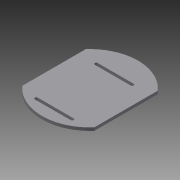
# Autodesk Inventor part: top
Saved by Autodesk Inventor 2015 (Build 190159000, 159)
## iProperties
Created: 2014-10-29
Part Number: top
Material: Generic
Document SubType Name: Modeling
Designer: Colin
Density: 1 g/cm^3
Appearance: Default
Author: Colin
Autodesk Inventor part; units mm, degrees
ref_plane "YZ Plane" through (0, 0, 0) normal (1, 0, 0) x (0, 1, 0)
ref_plane "XZ Plane" through (0, 0, 0) normal (0, 1, 0) x (-1, 0, 0)
ref_plane "XY Plane" through (0, 0, 0) normal (0, 0, 1) x (1, 0, 0)
sketch "Sketch1" plane through (0, 0, 0) normal (0, 1, 0) x (-1, 0, 0)
  arc A0 (38.1, 33.601) -> (-38.1, 33.601) centre (0, 0) ccw
  line L0 (38.1, -33.601) -> (38.1, 33.601)
  arc A1 (38.1, -33.601) -> (38.1, 33.601) centre (0, 0) ccw construction
  line L1 (-38.1, -33.601) -> (-38.1, 33.601)
  arc A2 (-38.1, -33.601) -> (38.1, -33.601) centre (0, 0) ccw
  arc A3 (-38.1, 33.601) -> (-38.1, -33.601) centre (0, 0) ccw construction
  dimension "d0" = 101.6
  dimension "d3" = 12.7
  dimension "d4" = 76.2
  constraints: 9 point on circle, 4 centre point, 4 end point, 2 vertical, 1 coincident
  measures "d0" diameter of A0
  measures "d3" distance edge to line of A0 L0
  measures "d4" distance between parallel lines of L0 L1
extrude "Extrusion1" add sketch "Sketch1" along normal blind 3.175
sketch "Sketch2" plane through (0, 3.175, 0) normal (0, 1, 0) x (1, 0, 0)
  line L0 (-38.1, 33.601) -> (38.1, 33.601) construction
  line L1 (38.1, -33.601) -> (-38.1, -33.601) construction
  line L2 (-38.1, -6.0865) -> (38.1, -6.0865) construction
  line L3 (38.1, 33.601) -> (38.1, -33.601) construction
  line L4 (38.1, -33.601) -> (38.1, 33.601) construction
  line L5 (-19.05, 27.251) -> (19.05, 27.251)
  line L6 (19.05, 24.076) -> (-19.05, 24.076)
  arc A0 (-19.05, 27.251) -> (-19.05, 24.076) centre (-19.05, 25.6635) ccw
  arc A1 (19.05, 24.076) -> (19.05, 27.251) centre (19.05, 25.6635) ccw
  line L7 (-38.1, 33.601) -> (-38.1, -33.601) projected
  line L8 (-19.05, -39.424) -> (19.05, -39.424)
  line L9 (19.05, -36.249) -> (-19.05, -36.249)
  arc A2 (-19.05, -36.249) -> (-19.05, -39.424) centre (-19.05, -37.8365) ccw
  arc A3 (19.05, -39.424) -> (19.05, -36.249) centre (19.05, -37.8365) ccw
  point P0 (0, 0)
  dimension "d11" = 19.05
  dimension "d12" = 19.05
  dimension "d13" = 6.35
  dimension "d14" = 3.175
  dimension "d17" = 63.5
  constraints: 16 end point, 8 point on circle, 6 symmetric about line, 4 centre point, 4 horizontal, 4 tangent, 2 equal length, 2 other
  measures "d11" distance from line of L7 A0.centre
  measures "d12" distance from line of L3 A1.centre
  measures "d13" distance between parallel lines of L0 L5
  measures "d14" distance between parallel lines of L5 L6
  measures "d17" distance of A0.centre A2.centre
extrude "Extrusion2" cut sketch "Sketch2" against normal through all
body "Solid1"
